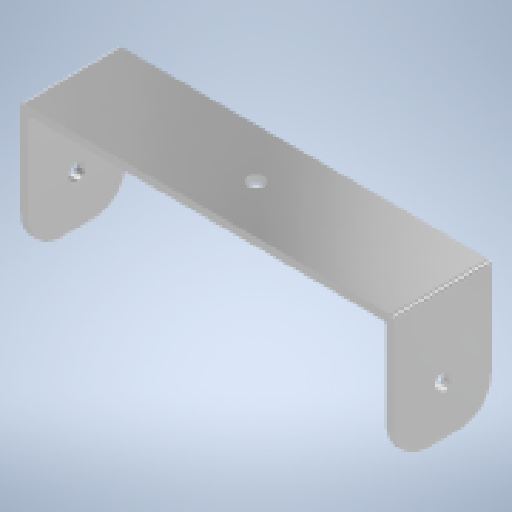
# Autodesk Inventor part: Bracket
Saved by Autodesk Inventor 2024 (Build 280153000, 153)
## iProperties
Created: 2023-10-06
Part Number: Bracket
Material: Aluminum 6061
Document SubType Name: Modeling
Designer: tangl
Density: 2.7 g/cm^3
Appearance: Aluminum - Flat
Author: tangl
Autodesk Inventor part; units mm, degrees
ref_plane "YZ Plane" through (0, 0, 0) normal (1, 0, 0) x (0, 1, 0)
ref_plane "XZ Plane" through (0, 0, 0) normal (0, 1, 0) x (-1, 0, 0)
ref_plane "XY Plane" through (0, 0, 0) normal (0, 0, 1) x (1, 0, 0)
sketch "Sketch1" plane through (0, 0, 0) normal (0, 1, 0) x (-1, 0, 0)
  line L0 (0, 0) -> (292.1, 0)
  line L1 (292.1, 0) -> (292.1, -76.2)
  line L2 (292.1, -76.2) -> (0, -76.2)
  line L3 (0, -76.2) -> (0, 0)
  circle A0 centre (146.05, -38.1) radius 6.35
  point P0 (292.1, -38.1)
  dimension "d0" = 292.1
  dimension "d1" = 76.2
  dimension "d27" = 12.7
  dimension "d28" = 38.1
  dimension "d45" = 146.05
  dimension "d46" = 146.05
  constraints: 8 end point, 3 perpendicular, 1 centre point, 1 horizontal, 1 midpoint
  measures "d0" distance of L0.start L0.end
  measures "d1" distance of L0.end L1.end
  measures "d27" diameter of A0
  measures "d28" distance from line of L0 A0.centre
  measures "d45" distance from line of L1 A0.centre
  measures "d46" distance from line of L3 A0.centre
extrude "Extrusion4" add sketch "Sketch1" along normal blind 101.6
sketch "Sketch4" plane through (-292.1, 0, 0) normal (0, 0, 1) x (1, 0, 0)
  line L0 (285.75, -50.8) -> (6.35, -50.8)
  line L1 (6.35, -50.8) -> (6.35, 95.25)
  line L2 (6.35, 95.25) -> (285.75, 95.25)
  line L3 (285.75, 95.25) -> (285.75, -50.8)
  line L4 (0, 101.6) -> (292.1, 101.6) projected
  line L5 (292.1, 0) -> (292.1, 101.6) projected
  line L6 (0, 0) -> (0, 101.6) projected
  point P0 (0, 50.8)
  dimension "d32" = 6.35
  dimension "d33" = 6.35
  dimension "d34" = 6.35
  dimension "d43" = 146.05
  constraints: 8 end point, 2 parallel, 1 horizontal, 1 midpoint, 1 perpendicular
  measures "d32" distance between parallel lines of L4 L2
  measures "d33" distance between parallel lines of L5 L3
  measures "d34" distance from line of point (0, 50.8) L1
  measures "d43" distance of L2.end L0.start
extrude "Extrusion5" cut sketch "Sketch4" against normal blind 119.0625
fillet "Fillet4" radius 25.4 4 edges at (-288.925, 0, 0) (-288.925, 0, -76.2) (-3.175, 0, 0) (-3.175, 0, -76.2)
sketch "Sketch5" plane through (0, 101.6, 0) normal (1, 0, 0) x (0, 0, -1)
  circle A0 centre (38.1, -63.5) radius 6.35
  line L0 (0, 0) -> (76.2, 0) projected
  line L1 (0, -76.2) -> (0, 0) projected
  point P0 (0, -101.6)
  dimension "d38" = 12.7
  dimension "d39" = 63.5
  dimension "d40" = 38.1
  constraints: 1 centre point
  measures "d38" diameter of A0
  measures "d39" distance from line of L0 A0.centre
  measures "d40" distance from line of L1 A0.centre
extrude "Extrusion6" cut sketch "Sketch5" against normal blind 330.2
fillet "Fillet5" radius 3.175 4 edges at (-292.1, 101.6, -38.1) (-285.75, 95.25, -38.1) (0, 101.6, -38.1) (-6.35, 95.25, -38.1)
body "Solid2"
